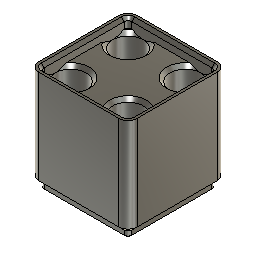
Magnet Dispenser Bin V2 (Autodesk Fusion 360 design; units mm, degrees)
Autodesk Fusion 360 part; units mm, degrees
note: some values were not read from the file. Set by a fixed rule: which face or edge a step refers to.
sketch "Sketch1" plane through (0, 0, 0) normal (0, 0, 1) x (1, 0, 0) in component "Gridfinity bin 1x1x1"
  line L0 (0, 0) -> (41.8, 0)
  line L1 (41.8, 0) -> (41.8, 41.8)
  line L2 (41.8, 41.8) -> (0, 41.8)
  line L3 (0, 41.8) -> (0, 0)
  dimension "d1" = 41.8
  dimension "d2" = 41.8
  constraint horizontal L0
  constraint vertical L1
  constraint horizontal L2
  constraint vertical L3
  constraint coincident L0.start L3
  constraint coincident L3.end L0
  measures "d1" horizontal distance of L0.start L0.end
  measures "d2" vertical distance of L0.end L1.end
extrude "Extrude1" add sketch "Sketch1" against normal blind 2.3 makes body 1 in component "Gridfinity bin 1x1x1"
fillet "Fillet1" radius 3.9 4 edges at (0, 0, -1.15) (41.8, 0, -1.15) (41.8, 41.8, -1.15) (0, 41.8, -1.15) on bodies 1 in component "Gridfinity bin 1x1x1"
chamfer "Chamfer1" distance 2.3 angle 45 8 edges at (1.1423, 40.6577, -2.3) (0, 20.9, -2.3) (1.1423, 1.1423, -2.3) (20.9, 0, -2.3) (40.6577, 1.1423, -2.3) (41.8, 20.9, -2.3) (40.6577, 40.6577, -2.3) (20.9, 41.8, -2.3) on bodies 1 in component "Gridfinity bin 1x1x1"
extrude "Extrude2" add 1 faces at (26.5667, 15.7668, -2.3) along direction (0, 0, -1) blind 2.7 on bodies 1 bodies 1 in component "Gridfinity bin 1x1x1"
chamfer "Chamfer2" distance 0.8 angle 45 8 edges at (2.7686, 39.0314, -5) (20.9, 39.5, -5) (39.0314, 39.0314, -5) (39.5, 20.9, -5) (39.0314, 2.7686, -5) (20.9, 2.3, -5) (2.7686, 2.7686, -5) (2.3, 20.9, -5) on bodies 1 in component "Gridfinity bin 1x1x1"
sketch "Sketch2" plane through (0, 0, -5) normal (0, 0, -1) x (-1, 0, 0) in component "Gridfinity bin 1x1x1"
  arc A0 (-3.1, 37.9) -> (-3.9, 38.7) centre (-3.9, 37.9) ccw construction
  line L0 (-3.9, 38.7) -> (-37.9, 38.7) construction
  arc A1 (-37.9, 38.7) -> (-38.7, 37.9) centre (-37.9, 37.9) ccw construction
  line L1 (-38.7, 37.9) -> (-38.7, 3.9) construction
  arc A2 (-38.7, 3.9) -> (-37.9, 3.1) centre (-37.9, 3.9) ccw construction
  line L2 (-37.9, 3.1) -> (-3.9, 3.1) construction
  arc A3 (-3.9, 3.1) -> (-3.1, 3.9) centre (-3.9, 3.9) ccw construction
  line L3 (-3.1, 3.9) -> (-3.1, 37.9) construction
  circle A4 centre (-8, 8) radius 3.25
  dimension "d11" = 6.5
  dimension "d12" = 8
  dimension "d13" = 8
  measures "d11" diameter of A4
  measures "d12" horizontal distance of origin A4.centre
  measures "d13" vertical distance of origin A4.centre
extrude "Extrude3" cut sketch "Sketch2" against normal blind 2.4 bodies 1 in component "Gridfinity bin 1x1x1"
pattern_linear "R-Pattern1" count 2 spacing 26 along (1, 0, 0) count 2 spacing 26 along (0, 1, 0) of "Extrude3" in component "Gridfinity bin 1x1x1"
pattern_linear "R-Pattern2" count 1 spacing 42 along (1, 0, 0) of bodies 1 merged in component "Gridfinity bin 1x1x1"
sketch "Sketch3" plane through (0, 0, 0) normal (0, 0, 1) x (1, 0, 0) in component "Gridfinity bin 1x1x1"
  line L0 (0, 0) -> (41.8, 0)
  line L1 (41.8, 0) -> (41.8, 41.8)
  line L2 (41.8, 41.8) -> (0, 41.8)
  line L3 (0, 41.8) -> (0, 0)
  dimension "d24" = 41.8
  dimension "d25" = 41.8
  constraint horizontal L0
  constraint vertical L1
  constraint horizontal L2
  constraint vertical L3
  constraint coincident L0.start L3
  constraint coincident L3.end L0
  measures "d24" horizontal distance of L0.start L0.end
  measures "d25" vertical distance of L0.end L1.end
extrude "Extrude4" add sketch "Sketch3" along normal blind 40 separate body makes body 2 in component "Gridfinity bin 1x1x1"
fillet "Fillet2" radius 3.9 8 edges at (0, 0, 20) (0, 41.8, 20) (0, 41.8, 20) (41.8, 41.8, 20) (41.8, 0, 20) (0, 0, 20) (41.8, 41.8, 20) (41.8, 0, 20) on bodies 2 in component "Gridfinity bin 1x1x1"
sketch "Sketch4" plane through (0, 0, 40) normal (0, 0, 1) x (1, 0, 0) in component "Gridfinity bin 1x1x1"
  arc A0 (37.9, 0) -> (41.8, 3.9) centre (37.9, 3.9) ccw construction
  line L0 (41.8, 3.9) -> (41.8, 37.9) construction
  arc A1 (41.8, 37.9) -> (37.9, 41.8) centre (37.9, 37.9) ccw construction
  line L1 (37.9, 41.8) -> (3.9, 41.8) construction
  arc A2 (3.9, 41.8) -> (0, 37.9) centre (3.9, 37.9) ccw construction
  line L2 (0, 37.9) -> (0, 3.9) construction
  arc A3 (0, 3.9) -> (3.9, 0) centre (3.9, 3.9) ccw construction
  line L3 (3.9, 0) -> (37.9, 0) construction
  arc A4 (37.9, 2.25) -> (39.55, 3.9) centre (37.9, 3.9) ccw
  line L4 (39.55, 3.9) -> (39.55, 37.9)
  arc A5 (39.55, 37.9) -> (37.9, 39.55) centre (37.9, 37.9) ccw
  line L5 (37.9, 39.55) -> (3.9, 39.55)
  arc A6 (3.9, 39.55) -> (2.25, 37.9) centre (3.9, 37.9) ccw
  line L6 (2.25, 37.9) -> (2.25, 3.9)
  arc A7 (2.25, 3.9) -> (3.9, 2.25) centre (3.9, 3.9) ccw
  line L7 (3.9, 2.25) -> (37.9, 2.25)
  dimension "d30" = -2.25
extrude "Extrude5" cut sketch "Sketch4" against normal blind 4 bodies 2 in component "Gridfinity bin 1x1x1"
chamfer "Chamfer3" distance 1.2 angle 45 8 edges at (39.55, 20.9, 40) (39.0667, 2.7333, 40) (20.9, 2.25, 40) (2.7333, 2.7333, 40) (2.25, 20.9, 40) (2.7333, 39.0667, 40) (20.9, 39.55, 40) (39.0667, 39.0667, 40) on bodies 2 in component "Gridfinity bin 1x1x1"
combine "Combine1" operation add target body 2 tool bodies 1 in component "Gridfinity bin 1x1x1"
sketch "Sketch6" plane through (0, 0, 36) normal (0, 0, 1) x (-1, 0, 0) in component "Gridfinity bin 1x1x1"
  line L0 (-3.9, -2.25) -> (-37.9, -2.25)
  arc A0 (-37.9, -2.25) -> (-39.55, -3.9) centre (-37.9, -3.9) ccw
  line L1 (-39.55, -3.9) -> (-39.55, -37.9)
  arc A1 (-39.55, -37.9) -> (-37.9, -39.55) centre (-37.9, -37.9) ccw
  line L2 (-37.9, -39.55) -> (-3.9, -39.55)
  arc A2 (-3.9, -39.55) -> (-2.25, -37.9) centre (-3.9, -37.9) ccw
  line L3 (-2.25, -37.9) -> (-2.25, -3.9)
  arc A3 (-2.25, -3.9) -> (-3.9, -2.25) centre (-3.9, -3.9) ccw
  arc A4 (-37.9, 0) -> (-41.8, -3.9) centre (-37.9, -3.9) ccw
  line L4 (-41.8, -3.9) -> (-41.8, -37.9)
  arc A5 (-41.8, -37.9) -> (-37.9, -41.8) centre (-37.9, -37.9) ccw
  line L5 (-37.9, -41.8) -> (-3.9, -41.8)
  arc A6 (-3.9, -41.8) -> (0, -37.9) centre (-3.9, -37.9) ccw
  line L6 (0, -37.9) -> (0, -3.9)
  arc A7 (0, -3.9) -> (-3.9, 0) centre (-3.9, -3.9) ccw
  line L7 (-3.9, 0) -> (-37.9, 0)
  line L8 (-40.75, -37.9) -> (-40.75, -3.9)
  arc A8 (-37.9, -1.05) -> (-40.75, -3.9) centre (-37.9, -3.9) ccw
  line L9 (-37.9, -1.05) -> (-3.9, -1.05)
  arc A9 (-1.05, -3.9) -> (-3.9, -1.05) centre (-3.9, -3.9) ccw
  line L10 (-1.05, -3.9) -> (-1.05, -37.9)
  arc A10 (-3.9, -40.75) -> (-1.05, -37.9) centre (-3.9, -37.9) ccw
  line L11 (-3.9, -40.75) -> (-37.9, -40.75)
  arc A11 (-40.75, -37.9) -> (-37.9, -40.75) centre (-37.9, -37.9) ccw
  circle A12 centre (-33.073, -8.727) radius 6.477
  circle A13 centre (-8.727, -8.727) radius 6.477
  circle A14 centre (-33.073, -33.073) radius 6.477
  circle A15 centre (-8.727, -33.073) radius 6.477
  dimension "d38" = 12.954
  dimension "d39" = 12.954
  dimension "d40" = 12.954
  dimension "d41" = 12.954
  constraint tangent L0 A12
  constraint tangent L1 A12
  constraint tangent L0 A13
  constraint tangent L3 A13
  constraint tangent L1 A14
  constraint tangent L2 A14
  constraint tangent L3 A15
  constraint tangent L2 A15
  measures "d38" diameter of A12
  measures "d39" diameter of A13
  measures "d40" diameter of A14
  measures "d41" diameter of A15
extrude "Extrude6" cut sketch "Sketch6" against normal up to surface (32.25 mm away) contours A13 | A12 | A15 | A14 bodies 2 in component "Gridfinity bin 1x1x1"
chamfer "Chamfer4" distance 1.397 angle 45 8 edges at (28.4931, 28.4931, 36) (37.6529, 37.6529, 36) (13.3069, 28.4931, 36) (4.1471, 37.6529, 36) (13.3069, 13.3069, 36) (4.1471, 4.1471, 36) (28.4931, 13.3069, 36) (37.6529, 4.1471, 36) on bodies 2 in component "Gridfinity bin 1x1x1"
component "Gridfinity bin 1x1x1" placed x (1, 0, 0) y (0, 1, 0) z (0, 0, 1) at (0, 0, 0)
equation "d3 = -( 2.30 mm )"
equation "d14 = -( 2.40 mm )"
equation "d31 = -( 4.00 mm )"
named bodies: "base", "Gridfinity bin 1x1x1"
